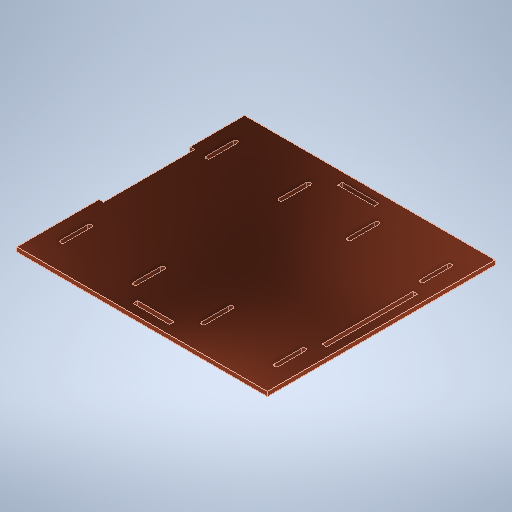
# Autodesk Inventor part: base_2
Saved by Autodesk Inventor 2025.3 (Build 293356030, 356C)
## iProperties
Created: 2026-06-26
Part Number: base_2
Material: Generic
Document SubType Name: Modeling
Designer: user
Density: 1 g/cm^3
Appearance: Copper - Polished
Author: user
Autodesk Inventor part; units mm, degrees
ref_plane "YZ Plane" through (0, 0, 0) normal (1, 0, 0) x (0, 1, 0)
ref_plane "XZ Plane" through (0, 0, 0) normal (0, 1, 0) x (-1, 0, 0)
ref_plane "XY Plane" through (0, 0, 0) normal (0, 0, 1) x (1, 0, 0)
sketch "Sketch1" plane through (0, 0, 0) normal (0, 1, 0) x (-1, 0, 0)
  line L0 (0, 0) -> (-275, 0)
  line L1 (-275, 0) -> (-275, -250)
  line L2 (-275, -250) -> (0, -250)
  line L3 (0, -250) -> (0, 0)
  line L4 (0, -125) -> (-275, -125) construction
  line L5 (-137.5, 0) -> (-137.5, -250) construction
  line L6 (-60, 0) -> (-60, -250) construction
  line L7 (-198, 0) -> (-198, -250) construction
  line L8 (-20, -220) -> (-20, -190) construction
  line L9 (-20, -220) -> (-20, -190) construction
  line L10 (-17.75, -220) -> (-17.75, -190)
  line L11 (-22.25, -190) -> (-22.25, -220)
  arc A0 (-22.25, -220) -> (-17.75, -220) centre (-20, -220) ccw
  arc A1 (-17.75, -190) -> (-22.25, -190) centre (-20, -190) ccw
  line L12 (-100, -220) -> (-100, -190) construction
  line L13 (-100, -220) -> (-100, -190) construction
  line L14 (-102.25, -220) -> (-102.25, -190)
  line L15 (-97.75, -190) -> (-97.75, -220)
  arc A2 (-102.25, -220) -> (-97.75, -220) centre (-100, -220) ccw
  arc A3 (-97.75, -190) -> (-102.25, -190) centre (-100, -190) ccw
  line L16 (-157.5, -240) -> (-117.5, -240)
  line L17 (-117.5, -240) -> (-117.5, -235)
  line L18 (-117.5, -235) -> (-157.5, -235)
  line L19 (-157.5, -235) -> (-157.5, -240)
  line L20 (-255, -220) -> (-255, -190) construction
  line L21 (-255, -220) -> (-255, -190) construction
  line L22 (-257.25, -220) -> (-257.25, -190)
  line L23 (-252.75, -190) -> (-252.75, -220)
  arc A4 (-257.25, -220) -> (-252.75, -220) centre (-255, -220) ccw
  arc A5 (-252.75, -190) -> (-257.25, -190) centre (-255, -190) ccw
  line L24 (-177.25, -190) -> (-177.25, -220)
  line L25 (-175, -220) -> (-175, -190) construction
  line L26 (-172.75, -220) -> (-172.75, -190)
  arc A6 (-177.25, -220) -> (-172.75, -220) centre (-175, -220) ccw
  line L27 (-175, -220) -> (-175, -190) construction
  arc A7 (-172.75, -190) -> (-177.25, -190) centre (-175, -190) ccw
  line L28 (-137.5, -250) -> (-137.5, 0) construction
  line L29 (-20, -30) -> (-20, -60) construction
  line L30 (-20, -30) -> (-20, -60) construction
  line L31 (-17.75, -30) -> (-17.75, -60)
  line L32 (-22.25, -60) -> (-22.25, -30)
  arc A8 (-17.75, -30) -> (-22.25, -30) centre (-20, -30) ccw
  arc A9 (-22.25, -60) -> (-17.75, -60) centre (-20, -60) ccw
  line L33 (-97.75, -60) -> (-97.75, -30)
  line L34 (-100, -30) -> (-100, -60) construction
  line L35 (-102.25, -30) -> (-102.25, -60)
  arc A10 (-97.75, -30) -> (-102.25, -30) centre (-100, -30) ccw
  line L36 (-100, -30) -> (-100, -60) construction
  arc A11 (-102.25, -60) -> (-97.75, -60) centre (-100, -60) ccw
  line L37 (-157.5, -10) -> (-117.5, -10)
  line L38 (-117.5, -10) -> (-117.5, -15)
  line L39 (-117.5, -15) -> (-157.5, -15)
  line L40 (-157.5, -15) -> (-157.5, -10)
  arc A12 (-252.75, -30) -> (-257.25, -30) centre (-255, -30) ccw
  line L41 (-252.75, -60) -> (-252.75, -30)
  line L42 (-255, -30) -> (-255, -60) construction
  line L43 (-255, -30) -> (-255, -60) construction
  arc A13 (-257.25, -60) -> (-252.75, -60) centre (-255, -60) ccw
  line L44 (-257.25, -30) -> (-257.25, -60)
  line L45 (-177.25, -60) -> (-177.25, -30)
  line L46 (-175, -30) -> (-175, -60) construction
  line L47 (-175, -30) -> (-175, -60) construction
  arc A14 (-177.25, -60) -> (-172.75, -60) centre (-175, -60) ccw
  line L48 (-172.75, -30) -> (-172.75, -60)
  arc A15 (-172.75, -30) -> (-177.25, -30) centre (-175, -30) ccw
  line L49 (-265, -102.5) -> (-265, -152.5)
  line L50 (-265, -152.5) -> (-265, -175)
  line L51 (-265, -175) -> (-260, -175)
  line L52 (-260, -175) -> (-260, -75)
  line L53 (-260, -75) -> (-265, -75)
  line L54 (-265, -75) -> (-265, -102.5)
  line L55 (0, -90) -> (-5, -90)
  line L56 (-5, -90) -> (-5, -190)
  line L57 (-5, -190) -> (0, -190)
  line L58 (0, -190) -> (0, -90)
  point P0 (-20, -205)
  point P1 (-100, -205)
  point P2 (-255, -205)
  point P3 (-175, -205)
  point P4 (-20, -45)
  point P5 (-100, -45)
  point P6 (-255, -45)
  point P7 (-175, -45)
  point P8 (0, -190)
  point P9 (-100, -205)
  point P10 (-20, -205)
  dimension "d2" = 30
  dimension "d4" = 30
  dimension "d6" = 2.25
  dimension "d9" = 40
  dimension "d13" = 10
  dimension "d14" = 5
  dimension "d16" = 20
  dimension "d21" = 5
  dimension "d22" = 5
  dimension "d26" = 50
  dimension "d27" = 50
  dimension "d28" = 10
  dimension "d30" = 250
  dimension "d31" = 275
  dimension "d32" = 80
  dimension "d33" = 20
  constraints: 134 end point, 55 symmetric about line, 32 point on circle, 16 centre point, 8 equal length, 7 midpoint, 6 point on line, 5 perpendicular, 4 tangent, 3 horizontal, 1 vertical, 14 other
  measures "d2" distance of L8.start L8.end
  measures "d4" distance from line of L2 L8.start
  measures "d6" radius of A0
  measures "d9" distance of L18.end L17.end
  measures "d13" distance between parallel lines of L2 L16
  measures "d14" distance between parallel lines of L18 L16
  measures "d16" distance between parallel lines of L5 L19
  measures "d21" distance of L57.end L56.end
  measures "d22" distance between parallel lines of L50 L52
  measures "d26" distance between parallel lines of L4 L53
  measures "d27" distance between parallel lines of L4 L51
  measures "d28" distance between parallel lines of L1 L49
  measures "d30" distance between parallel lines of L0 L2
  measures "d31" distance between parallel lines of L3 L1
  measures "d32" distance of point (-100, -205) point (-20, -205)
  measures "d33" distance from line of L3 point (-20, -205)
extrude "Extrusion1" add sketch "Sketch1" along normal blind 5 contours L3 L55 L56 L57 L2 L1 L0
body "Solid1"
